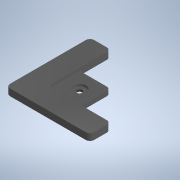
# Autodesk Inventor part: Standoff_Corner
Saved by Autodesk Inventor 2022 (Build 260153000, 153)
## iProperties
Part Number: Standoff_Corner
Material: Generic
Document SubType Name: Modeling
Designer: braxt
Appearance: Default
Author: braxt
Autodesk Inventor part; units mm, degrees
ref_plane "YZ Plane" through (0, 0, 0) normal (1, 0, 0) x (0, 1, 0)
ref_plane "XZ Plane" through (0, 0, 0) normal (0, 1, 0) x (-1, 0, 0)
ref_plane "XY Plane" through (0, 0, 0) normal (0, 0, 1) x (1, 0, 0)
sketch "Sketch1" plane through (0, 0, 0) normal (0, 1, 0) x (-1, 0, 0)
  line L0 (0, -2) -> (0, -38)
  line L1 (-2, 0) -> (-38, 0)
  line L2 (-40, -2) -> (-40, -8)
  line L3 (-38, -10) -> (-27, -10)
  line L4 (-10, -27) -> (-10, -38)
  line L5 (-8, -40) -> (-2, -40)
  line L6 (-12, -25) -> (-23, -25)
  line L7 (-25, -23) -> (-25, -12)
  arc A0 (-10, -27) -> (-12, -25) centre (-12, -27) ccw
  arc A1 (-25, -23) -> (-23, -25) centre (-23, -23) ccw
  arc A2 (-25, -12) -> (-27, -10) centre (-27, -12) ccw
  arc A3 (-10, -38) -> (-8, -40) centre (-8, -38) ccw
  arc A4 (-40, -8) -> (-38, -10) centre (-38, -8) ccw
  arc A5 (-38, 0) -> (-40, -2) centre (-38, -2) ccw
  arc A6 (0, -2) -> (-2, 0) centre (-2, -2) ccw
  arc A7 (-2, -40) -> (0, -38) centre (-2, -38) ccw
  line L8 (-27, -10) -> (-12, -10)
  line L9 (-10, -27) -> (-10, -12)
  arc A8 (-10, -12) -> (-12, -10) centre (-12, -12) ccw
  point P0 (0, 0)
  point P1 (0, -40)
  point P2 (-40, 0)
  point P3 (-40, -10)
  point P4 (-10, -10)
  point P5 (-10, -40)
  point P6 (-10, -25)
  point P7 (-25, -25)
  point P8 (-25, -10)
  point P9 (-17.5, -17.5)
  dimension "d0" = 40
  dimension "d2" = 10
  dimension "d8" = 15
  dimension "d9" = 15
  dimension "d11" = 10
  dimension "d12" = 40
  dimension "d13" = 2
  dimension "d14" = 2
  constraints: 20 end point, 20 point on line, 19 point on circle, 18 tangent, 9 centre point, 7 equal radius, 7 perpendicular, 2 horizontal, 1 vertical
  measures "d0" distance of point (0, 0) point (0, -40)
  measures "d2" distance of point (-40, 0) point (-40, -10)
  measures "d8" distance of point (-10, -25) point (-25, -25)
  measures "d9" distance of point (-25, -25) point (-25, -10)
  measures "d11" distance of point (-10, -40) point (0, -40)
  measures "d12" distance of point (0, 0) point (-40, 0)
  measures "d13" radius of A0
  measures "d14" radius of A8
extrude "Extrusion1" add sketch "Sketch1" along normal blind 1.175 contours L0 A7 L5 A3 L4 L9 A8 L8 L3 A4 L2 A5 L1 A6
extrude "Extrusion2" add sketch "Sketch1" against normal blind 2
hole "Hole1" at (17.5, 0, -17.5) direction (0, -1, 0) diameter 2.459 depth 8.8 tip angle 118 counterbore diameter 6 counterbore depth 1 thread size "M3x0.5" class "6H" standard "ANSI Metric M Profile"
body "Solid1"
